Autodesk Inventor part; units mm, degrees
(part 3 of 8)
sketch "20" plane through (0, 0, 0) normal (0, 0, 1) x (1, 0, 0)
  line L0 (110.47, 0) -> (110.47, 86.411)
  line L1 (110.47, 86.411) -> (0, 86.411)
  line L2 (0, 86.411) -> (0, 0)
  line L3 (-2.54, 0) -> (-10.84, 0)
  arc A0 (-10.84, 0.0325) -> (-10.84, -0.0325) centre (-10.84, 0) ccw
  arc A1 (-2.54, -0.0325) -> (-2.54, 0.0325) centre (-2.54, 0) ccw
  line L4 (-2.54, 85.09) -> (-10.84, 85.09)
  arc A2 (-10.84, 85.1225) -> (-10.84, 85.0575) centre (-10.84, 85.09) ccw
  arc A3 (-2.54, 85.0575) -> (-2.54, 85.1225) centre (-2.54, 85.09) ccw
  line L5 (-8.89, 0.065) -> (-8.89, 85.025)
  arc A4 (-8.8575, 85.025) -> (-8.9225, 85.025) centre (-8.89, 85.025) ccw
  arc A5 (-8.9225, 0.065) -> (-8.8575, 0.065) centre (-8.89, 0.065) ccw
  line L6 (-8.89, 0.065) -> (-9.2092, 2.6)
  arc A6 (-9.177, 2.6041) -> (-9.2415, 2.5959) centre (-9.2093, 2.6) ccw
  arc A7 (-8.9222, 0.0609) -> (-8.8578, 0.0691) centre (-8.89, 0.065) ccw
  line L7 (-9.2092, 2.6) -> (-8.5708, 2.6)
  arc A8 (-8.5708, 2.5675) -> (-8.5708, 2.6325) centre (-8.5708, 2.6) ccw
  arc A9 (-9.2092, 2.6325) -> (-9.2092, 2.5675) centre (-9.2092, 2.6) ccw
  line L8 (-8.5708, 2.6) -> (-8.89, 0.065)
  arc A10 (-8.9222, 0.0691) -> (-8.8578, 0.0609) centre (-8.89, 0.065) ccw
  arc A11 (-8.5385, 2.5959) -> (-8.603, 2.6041) centre (-8.5707, 2.6) ccw
  line L9 (-8.89, 0.065) -> (-9.02, 2.6)
  arc A12 (-8.9875, 2.6017) -> (-9.0525, 2.5983) centre (-9.02, 2.6) ccw
  arc A13 (-8.9225, 0.0633) -> (-8.8575, 0.0667) centre (-8.89, 0.065) ccw
  line L10 (-8.76, 2.6) -> (-8.89, 0.065)
  arc A14 (-8.9225, 0.0667) -> (-8.8575, 0.0633) centre (-8.89, 0.065) ccw
  arc A15 (-8.7275, 2.5983) -> (-8.7925, 2.6017) centre (-8.76, 2.6) ccw
  line L11 (-8.89, 0.065) -> (-9.15, 2.6)
  arc A16 (-9.1177, 2.6033) -> (-9.1823, 2.5967) centre (-9.15, 2.6) ccw
  arc A17 (-8.9223, 0.0617) -> (-8.8577, 0.0683) centre (-8.89, 0.065) ccw
  line L12 (-8.63, 2.6) -> (-8.89, 0.065)
  arc A18 (-8.9223, 0.0683) -> (-8.8577, 0.0617) centre (-8.89, 0.065) ccw
  arc A19 (-8.5977, 2.5967) -> (-8.6623, 2.6033) centre (-8.63, 2.6) ccw
  line L13 (-8.89, 85.025) -> (-9.2092, 82.49)
  arc A20 (-9.2415, 82.4941) -> (-9.177, 82.4859) centre (-9.2093, 82.49) ccw
  arc A21 (-8.8578, 85.0209) -> (-8.9222, 85.0291) centre (-8.89, 85.025) ccw
  line L14 (-9.2092, 82.49) -> (-8.5708, 82.49)
  arc A22 (-8.5708, 82.4575) -> (-8.5708, 82.5225) centre (-8.5708, 82.49) ccw
  arc A23 (-9.2092, 82.5225) -> (-9.2092, 82.4575) centre (-9.2092, 82.49) ccw
  line L15 (-8.5708, 82.49) -> (-8.89, 85.025)
  arc A24 (-8.8578, 85.0291) -> (-8.9222, 85.0209) centre (-8.89, 85.025) ccw
  arc A25 (-8.603, 82.4859) -> (-8.5385, 82.4941) centre (-8.5707, 82.49) ccw
  line L16 (-8.89, 85.025) -> (-9.02, 82.49)
  arc A26 (-9.0525, 82.4917) -> (-8.9875, 82.4883) centre (-9.02, 82.49) ccw
  arc A27 (-8.8575, 85.0233) -> (-8.9225, 85.0267) centre (-8.89, 85.025) ccw
  line L17 (-8.76, 82.49) -> (-8.89, 85.025)
  arc A28 (-8.8575, 85.0267) -> (-8.9225, 85.0233) centre (-8.89, 85.025) ccw
  arc A29 (-8.7925, 82.4883) -> (-8.7275, 82.4917) centre (-8.76, 82.49) ccw
  line L18 (-8.89, 85.025) -> (-9.15, 82.49)
  arc A30 (-9.1823, 82.4933) -> (-9.1177, 82.4867) centre (-9.15, 82.49) ccw
  arc A31 (-8.8577, 85.0217) -> (-8.9223, 85.0283) centre (-8.89, 85.025) ccw
  line L19 (-8.63, 82.49) -> (-8.89, 85.025)
  arc A32 (-8.8577, 85.0283) -> (-8.9223, 85.0217) centre (-8.89, 85.025) ccw
  arc A33 (-8.6623, 82.4867) -> (-8.5977, 82.4933) centre (-8.63, 82.49) ccw
  arc A34 (-9.9923, 40.3333) -> (-9.9923, 39.4302) centre (-9.9923, 39.8817) ccw
  arc A35 (-9.9923, 40.2952) -> (-9.9923, 40.3714) centre (-9.9923, 40.3333) ccw
  arc A36 (-9.9923, 39.3921) -> (-9.9923, 39.4683) centre (-9.9923, 39.4302) ccw
  arc A37 (-9.9923, 39.4302) -> (-9.9923, 40.3333) centre (-9.9923, 39.8817) ccw
  arc A38 (-9.9923, 39.4683) -> (-9.9923, 39.3921) centre (-9.9923, 39.4302) ccw
  arc A39 (-9.9923, 40.3714) -> (-9.9923, 40.2952) centre (-9.9923, 40.3333) ccw
  arc A40 (-10.8051, 40.243) -> (-10.8051, 39.5205) centre (-10.8051, 39.8817) ccw
  arc A41 (-10.8051, 40.2049) -> (-10.8051, 40.2811) centre (-10.8051, 40.243) ccw
  arc A42 (-10.8051, 39.4824) -> (-10.8051, 39.5586) centre (-10.8051, 39.5205) ccw
  arc A43 (-10.8051, 39.5205) -> (-10.8051, 40.243) centre (-10.8051, 39.8817) ccw
  arc A44 (-10.8051, 39.5586) -> (-10.8051, 39.4824) centre (-10.8051, 39.5205) ccw
  arc A45 (-10.8051, 40.2811) -> (-10.8051, 40.2049) centre (-10.8051, 40.243) ccw
  line L20 (-9.5407, 40.9933) -> (-9.5407, 41.5352)
  arc A46 (-9.5026, 41.5352) -> (-9.5788, 41.5352) centre (-9.5407, 41.5352) ccw
  arc A47 (-9.5788, 40.9933) -> (-9.5026, 40.9933) centre (-9.5407, 40.9933) ccw
  arc A48 (-9.5407, 41.5352) -> (-9.9019, 41.8964) centre (-9.9019, 41.5352) ccw
  arc A49 (-9.5788, 41.5352) -> (-9.5026, 41.5352) centre (-9.5407, 41.5352) ccw
  arc A50 (-9.9019, 41.9345) -> (-9.9019, 41.8583) centre (-9.9019, 41.8964) ccw
  line L21 (-9.9019, 41.8964) -> (-10.0826, 41.8964)
  arc A51 (-10.0826, 41.9345) -> (-10.0826, 41.8583) centre (-10.0826, 41.8964) ccw
  arc A52 (-9.9019, 41.8583) -> (-9.9019, 41.9345) centre (-9.9019, 41.8964) ccw
  arc A53 (-10.0826, 41.8964) -> (-10.4438, 41.5352) centre (-10.0826, 41.5352) ccw
  arc A54 (-10.0826, 41.8583) -> (-10.0826, 41.9345) centre (-10.0826, 41.8964) ccw
  line L22 (110.425, 90.17) -> (107.89, 90.43)
  arc A55 (107.8883, 90.0725) -> (107.8917, 90.0075) centre (107.89, 90.04) ccw
  arc A56 (110.4267, 90.1375) -> (110.4233, 90.2025) centre (110.425, 90.17) ccw
  line L23 (107.89, 90.04) -> (110.425, 90.17)
  arc A57 (110.4233, 90.1375) -> (110.4267, 90.2025) centre (110.425, 90.17) ccw
  arc A58 (107.8917, 90.3325) -> (107.8883, 90.2675) centre (107.89, 90.3) ccw
  line L24 (110.425, 90.17) -> (107.89, 90.3)
  arc A59 (107.8859, 89.883) -> (107.8941, 89.8185) centre (107.89, 89.8507) ccw
  arc A60 (110.4291, 90.1378) -> (110.4209, 90.2022) centre (110.425, 90.17) ccw
  line L25 (107.89, 89.8508) -> (110.425, 90.17)
  arc A61 (58.3921, 91.9044) -> (58.7533, 91.5432) centre (58.7533, 91.9044) ccw
  arc A62 (59.2952, 91.5051) -> (59.2952, 91.5813) centre (59.2952, 91.5432) ccw
  arc A63 (58.7533, 91.5813) -> (58.7533, 91.5051) centre (58.7533, 91.5432) ccw
  line L26 (59.2952, 91.5432) -> (58.7533, 91.5432)
  arc A64 (2.6325, 90.4892) -> (2.5675, 90.4892) centre (2.6, 90.4892) ccw
  arc A65 (2.5675, 89.8508) -> (2.6325, 89.8508) centre (2.6, 89.8508) ccw
  line L27 (2.6, 90.4892) -> (2.6, 89.8508)
  arc A66 (0.0609, 90.2022) -> (0.0691, 90.1378) centre (0.065, 90.17) ccw
  arc A67 (2.6041, 90.457) -> (2.5959, 90.5215) centre (2.6, 90.4893) ccw
  line L28 (0.065, 90.17) -> (2.6, 90.4892)
  arc A68 (0.065, 90.2025) -> (0.065, 90.1375) centre (0.065, 90.17) ccw
  arc A69 (110.425, 90.1375) -> (110.425, 90.2025) centre (110.425, 90.17) ccw
  line L29 (0.065, 90.17) -> (110.425, 90.17)
  arc A70 (110.4575, 87.63) -> (110.5225, 87.63) centre (110.49, 87.63) ccw
  arc A71 (110.5225, 92.12) -> (110.4575, 92.12) centre (110.49, 92.12) ccw
  line L30 (110.49, 87.63) -> (110.49, 92.12)
  arc A72 (57.4992, 91.5432) -> (57.423, 91.5432) centre (57.4611, 91.5432) ccw
  arc A73 (57.423, 90.8207) -> (57.4992, 90.8207) centre (57.4611, 90.8207) ccw
  line L31 (57.4611, 91.5432) -> (57.4611, 90.8207)
  arc A74 (56.8289, 91.22) -> (56.8289, 91.1438) centre (56.8289, 91.1819) ccw
  arc A75 (57.732, 91.1438) -> (57.732, 91.22) centre (57.732, 91.1819) ccw
  line L32 (56.8289, 91.1819) -> (57.732, 91.1819)
  arc A76 (57.2268, 92.4358) -> (57.1535, 92.4568) centre (57.1902, 92.4463) ccw
  arc A77 (56.7923, 91.1924) -> (56.8656, 91.1715) centre (56.829, 91.182) ccw
  line L33 (59.2952, 91.9947) -> (59.2952, 91.5432)
  arc A78 (58.354, 91.9947) -> (58.4302, 91.9947) centre (58.3921, 91.9947) ccw
  arc A79 (59.2571, 91.9947) -> (59.3333, 91.9947) centre (59.2952, 91.9947) ccw
  arc A80 (107.8575, 89.8508) -> (107.9225, 89.8508) centre (107.89, 89.8508) ccw
  arc A81 (59.2952, 91.9947) -> (58.3921, 91.9947) centre (58.8436, 91.9947) ccw
  arc A82 (58.354, 91.9044) -> (58.4302, 91.9044) centre (58.3921, 91.9044) ccw
  arc A83 (58.4302, 91.9947) -> (58.354, 91.9947) centre (58.3921, 91.9947) ccw
  circle A84 centre (87.376, 65.7225) radius 1.524
  circle A85 centre (87.376, 19.431) radius 1.524
  circle A86 centre (22.225, 19.431) radius 1.524
  line L34 (57.1902, 92.4463) -> (56.8289, 91.1819)
  arc A87 (56.2315, 90.7826) -> (56.2315, 90.8588) centre (56.2315, 90.8207) ccw
  arc A88 (56.1411, 90.8588) -> (56.1411, 90.7826) centre (56.1411, 90.8207) ccw
  arc A89 (-0.0325, 87.63) -> (0.0325, 87.63) centre (0, 87.63) ccw
  arc A90 (0.0325, 92.12) -> (-0.0325, 92.12) centre (0, 92.12) ccw
  line L35 (0, 87.63) -> (0, 92.12)
  arc A91 (-10.2632, 45.686) -> (-10.2632, 45.6098) centre (-10.2632, 45.6479) ccw
  arc A92 (-9.5788, 44.9254) -> (-9.5026, 44.9254) centre (-9.5407, 44.9254) ccw
  arc A93 (-9.5407, 44.9254) -> (-10.2632, 45.6479) centre (-10.2632, 44.9254) ccw
  arc A94 (-10.7147, 45.686) -> (-10.7147, 45.6098) centre (-10.7147, 45.6479) ccw
  arc A95 (-10.2632, 45.6098) -> (-10.2632, 45.686) centre (-10.2632, 45.6479) ccw
  line L36 (-10.7147, 45.6479) -> (-10.2632, 45.6479)
  line L37 (56.2315, 90.8207) -> (56.1411, 90.8207)
  arc A96 (56.2696, 90.911) -> (56.1934, 90.911) centre (56.2315, 90.911) ccw
  arc A97 (56.1934, 90.8207) -> (56.2696, 90.8207) centre (56.2315, 90.8207) ccw
  line L38 (56.2315, 90.911) -> (56.2315, 90.8207)
  arc A98 (56.1411, 90.9491) -> (56.1411, 90.8729) centre (56.1411, 90.911) ccw
  arc A99 (56.2315, 90.8729) -> (56.2315, 90.9491) centre (56.2315, 90.911) ccw
  line L39 (56.1411, 90.911) -> (56.2315, 90.911)
  arc A100 (56.103, 90.8207) -> (56.1792, 90.8207) centre (56.1411, 90.8207) ccw
  arc A101 (56.1792, 90.911) -> (56.103, 90.911) centre (56.1411, 90.911) ccw
  line L40 (56.1411, 90.8207) -> (56.1411, 90.911)
  circle A102 centre (22.225, 65.7225) radius 1.524
  arc A103 (59.3333, 91.5432) -> (59.2571, 91.5432) centre (59.2952, 91.5432) ccw
  arc A104 (58.5727, 90.8588) -> (58.5727, 90.7826) centre (58.5727, 90.8207) ccw
  arc A105 (58.5727, 90.8207) -> (59.2952, 91.5432) centre (58.5727, 91.5432) ccw
  arc A106 (59.3333, 91.9947) -> (59.2571, 91.9947) centre (59.2952, 91.9947) ccw
  arc A107 (59.2571, 91.5432) -> (59.3333, 91.5432) centre (59.2952, 91.5432) ccw
  arc A108 (54.7011, 91.2057) -> (54.7606, 91.1581) centre (54.7309, 91.1819) ccw
  arc A109 (55.4831, 92.0613) -> (55.4236, 92.1089) centre (55.4534, 92.0851) ccw
  line L41 (54.7309, 91.1819) -> (55.4534, 92.0851)
  arc A110 (55.4442, 91.0341) -> (55.3722, 91.0588) centre (55.4082, 91.0464) ccw
  arc A111 (55.0921, 90.8588) -> (55.0921, 90.7826) centre (55.0921, 90.8207) ccw
  arc A112 (55.0921, 90.8207) -> (55.4082, 91.0465) centre (55.0921, 91.1548) ccw
  arc A113 (55.5818, 91.6335) -> (55.5056, 91.6335) centre (55.5437, 91.6335) ccw
  arc A114 (55.374, 91.0632) -> (55.4425, 91.0298) centre (55.4083, 91.0465) ccw
  arc A115 (55.4082, 91.0465) -> (55.5437, 91.6335) centre (54.2043, 91.6336) ccw
  arc A116 (55.0921, 90.7826) -> (55.0921, 90.8588) centre (55.0921, 90.8207) ccw
  arc A117 (54.8121, 91.0588) -> (54.74, 91.0341) centre (54.7761, 91.0464) ccw
  arc A118 (54.776, 91.0465) -> (55.0921, 90.8207) centre (55.0921, 91.1548) ccw
  arc A119 (54.7418, 91.0298) -> (54.8103, 91.0632) centre (54.7761, 91.0465) ccw
  arc A120 (54.6787, 91.6335) -> (54.6025, 91.6335) centre (54.6406, 91.6335) ccw
  arc A121 (54.6406, 91.6335) -> (54.776, 91.0465) centre (55.98, 91.6333) ccw
  arc A122 (55.4425, 92.2372) -> (55.374, 92.2038) centre (55.4083, 92.2205) ccw
  arc A123 (55.5056, 91.6335) -> (55.5818, 91.6335) centre (55.5437, 91.6335) ccw
  arc A124 (55.5437, 91.6335) -> (55.4082, 92.2205) centre (54.2043, 91.6334) ccw
  arc A125 (55.0921, 92.4844) -> (55.0921, 92.4082) centre (55.0921, 92.4463) ccw
  arc A126 (55.3722, 92.2082) -> (55.4442, 92.2329) centre (55.4082, 92.2206) ccw
  line L42 (0, 0) -> (110.47, 0)
  arc A127 (55.4082, 92.2205) -> (55.0921, 92.4463) centre (55.0921, 92.1122) ccw
  arc A128 (54.74, 92.2329) -> (54.8121, 92.2082) centre (54.7761, 92.2206) ccw
  arc A129 (55.0921, 92.4082) -> (55.0921, 92.4844) centre (55.0921, 92.4463) ccw
  arc A130 (55.0921, 92.4463) -> (54.776, 92.2205) centre (55.0921, 92.1122) ccw
  arc A131 (54.6025, 91.6335) -> (54.6787, 91.6335) centre (54.6406, 91.6335) ccw
  arc A132 (54.8103, 92.2038) -> (54.7418, 92.2372) centre (54.7761, 92.2205) ccw
  arc A133 (54.776, 92.2205) -> (54.6406, 91.6335) centre (55.98, 91.6337) ccw
  arc A134 (53.0774, 90.8588) -> (53.0774, 90.7826) centre (53.0774, 90.8207) ccw
  arc A135 (53.9805, 90.7826) -> (53.9805, 90.8588) centre (53.9805, 90.8207) ccw
  line L43 (53.0774, 90.8207) -> (53.9805, 90.8207)
  line L44 (107.89, 90.4892) -> (107.89, 89.8508)
  arc A136 (110.4209, 90.1378) -> (110.4291, 90.2022) centre (110.425, 90.17) ccw
  arc A137 (107.8941, 90.5215) -> (107.8859, 90.457) centre (107.89, 90.4893) ccw
  line L45 (110.425, 90.17) -> (107.89, 90.4892)
  arc A138 (2.5967, 89.8777) -> (2.6033, 89.9423) centre (2.6, 89.91) ccw
  arc A139 (0.0683, 90.2023) -> (0.0617, 90.1377) centre (0.065, 90.17) ccw
  line L46 (2.6, 89.91) -> (0.065, 90.17)
  arc A140 (0.0617, 90.2023) -> (0.0683, 90.1377) centre (0.065, 90.17) ccw
  arc A141 (2.6033, 90.3977) -> (2.5967, 90.4623) centre (2.6, 90.43) ccw
  line L47 (0.065, 90.17) -> (2.6, 90.43)
  arc A142 (2.5983, 90.0075) -> (2.6017, 90.0725) centre (2.6, 90.04) ccw
  arc A143 (0.0667, 90.2025) -> (0.0633, 90.1375) centre (0.065, 90.17) ccw
  line L48 (2.6, 90.04) -> (0.065, 90.17)
  arc A144 (0.0633, 90.2025) -> (0.0667, 90.1375) centre (0.065, 90.17) ccw
  arc A145 (2.6017, 90.2675) -> (2.5983, 90.3325) centre (2.6, 90.3) ccw
  line L49 (0.065, 90.17) -> (2.6, 90.3)
  arc A146 (2.5959, 89.8185) -> (2.6041, 89.883) centre (2.6, 89.8507) ccw
  arc A147 (0.0691, 90.2022) -> (0.0609, 90.1378) centre (0.065, 90.17) ccw
  arc A148 (53.5671, 92.4463) -> (53.4909, 92.4463) centre (53.529, 92.4463) ccw
  arc A149 (53.4909, 90.8207) -> (53.5671, 90.8207) centre (53.529, 90.8207) ccw
  line L50 (53.529, 92.4463) -> (53.529, 90.8207)
  line L51 (2.6, 89.8508) -> (0.065, 90.17)
  arc A150 (53.0536, 92.1148) -> (53.1012, 92.0553) centre (53.0774, 92.0851) ccw
  arc A151 (53.5528, 92.4165) -> (53.5052, 92.4761) centre (53.529, 92.4463) ccw
  line L52 (53.0774, 92.0851) -> (53.529, 92.4463)
  arc A152 (51.5143, 90.8588) -> (51.5143, 90.7826) centre (51.5143, 90.8207) ccw
  arc A153 (52.4174, 90.7826) -> (52.4174, 90.8588) centre (52.4174, 90.8207) ccw
  line L53 (51.5143, 90.8207) -> (52.4174, 90.8207)
  arc A154 (52.004, 92.4463) -> (51.9278, 92.4463) centre (51.9659, 92.4463) ccw
  arc A155 (107.9225, 90.4892) -> (107.8575, 90.4892) centre (107.89, 90.4892) ccw
  arc A156 (51.9278, 90.8207) -> (52.004, 90.8207) centre (51.9659, 90.8207) ccw
  line L54 (51.9659, 92.4463) -> (51.9659, 90.8207)
  arc A157 (51.4905, 92.1148) -> (51.5381, 92.0553) centre (51.5143, 92.0851) ccw
  arc A158 (51.9897, 92.4165) -> (51.9421, 92.4761) centre (51.9659, 92.4463) ccw
  line L55 (51.5143, 92.0851) -> (51.9659, 92.4463)
  arc A159 (107.8867, 89.9423) -> (107.8933, 89.8777) centre (107.89, 89.91) ccw
  arc A160 (110.4283, 90.1377) -> (110.4217, 90.2023) centre (110.425, 90.17) ccw
  line L56 (58.3921, 91.9044) -> (58.3921, 91.9947)
  arc A161 (58.7533, 91.5051) -> (58.7533, 91.5813) centre (58.7533, 91.5432) ccw
  arc A162 (58.4302, 91.9044) -> (58.354, 91.9044) centre (58.3921, 91.9044) ccw
  line L57 (107.89, 89.91) -> (110.425, 90.17)
  arc A163 (110.4217, 90.1377) -> (110.4283, 90.2023) centre (110.425, 90.17) ccw
  arc A164 (-10.7147, 44.7067) -> (-10.7147, 44.7829) centre (-10.7147, 44.7448) ccw
  arc A165 (-10.7147, 45.6098) -> (-10.7147, 45.686) centre (-10.7147, 45.6479) ccw
  arc A166 (-10.7147, 45.6479) -> (-10.7147, 44.7448) centre (-10.7147, 45.1964) ccw
  arc A167 (-10.6244, 44.7067) -> (-10.6244, 44.7829) centre (-10.6244, 44.7448) ccw
  arc A168 (-10.7147, 44.7829) -> (-10.7147, 44.7067) centre (-10.7147, 44.7448) ccw
  line L58 (-10.6244, 44.7448) -> (-10.7147, 44.7448)
  arc A169 (-10.2251, 45.1061) -> (-10.3013, 45.1061) centre (-10.2632, 45.1061) ccw
  arc A170 (-10.6244, 44.7829) -> (-10.6244, 44.7067) centre (-10.6244, 44.7448) ccw
  arc A171 (-10.6244, 44.7448) -> (-10.2632, 45.1061) centre (-10.6245, 45.1061) ccw
  arc A172 (-10.2251, 45.6479) -> (-10.3013, 45.6479) centre (-10.2632, 45.6479) ccw
  arc A173 (-10.3013, 45.1061) -> (-10.2251, 45.1061) centre (-10.2632, 45.1061) ccw
  line L59 (-10.2632, 45.6479) -> (-10.2632, 45.1061)
  arc A174 (-9.9257, 43.2422) -> (-9.8781, 43.3018) centre (-9.9019, 43.272) ccw
  arc A175 (-10.7813, 44.0242) -> (-10.8289, 43.9647) centre (-10.8051, 43.9945) ccw
  line L60 (-9.9019, 43.272) -> (-10.8051, 43.9945)
  arc A176 (-9.7541, 43.9854) -> (-9.7788, 43.9133) centre (-9.7664, 43.9493) ccw
  arc A177 (-9.5788, 43.6332) -> (-9.5026, 43.6332) centre (-9.5407, 43.6332) ccw
  arc A178 (-9.5407, 43.6332) -> (-9.7665, 43.9493) centre (-9.8748, 43.6332) ccw
  arc A179 (-10.3535, 44.1229) -> (-10.3535, 44.0467) centre (-10.3535, 44.0848) ccw
  arc A180 (-9.7832, 43.9151) -> (-9.7498, 43.9836) centre (-9.7665, 43.9494) ccw
  arc A181 (-9.7665, 43.9493) -> (-10.3535, 44.0848) centre (-10.3536, 42.7454) ccw
  arc A182 (-9.5026, 43.6332) -> (-9.5788, 43.6332) centre (-9.5407, 43.6332) ccw
  arc A183 (-9.7788, 43.3532) -> (-9.7541, 43.2811) centre (-9.7664, 43.3171) ccw
  arc A184 (-9.7665, 43.3172) -> (-9.5407, 43.6332) centre (-9.8748, 43.6332) ccw
  arc A185 (-9.7498, 43.2829) -> (-9.7832, 43.3514) centre (-9.7665, 43.3171) ccw
  arc A186 (-10.3535, 43.2198) -> (-10.3535, 43.1436) centre (-10.3535, 43.1817) ccw
  arc A187 (-10.3535, 43.1817) -> (-9.7665, 43.3172) centre (-10.3536, 44.5211) ccw
  arc A188 (-10.9572, 43.9836) -> (-10.9238, 43.9151) centre (-10.9405, 43.9494) ccw
  arc A189 (-10.3535, 44.0467) -> (-10.3535, 44.1229) centre (-10.3535, 44.0848) ccw
  arc A190 (-10.3535, 44.0848) -> (-10.9405, 43.9493) centre (-10.3534, 42.7454) ccw
  arc A191 (-11.2044, 43.6332) -> (-11.1282, 43.6332) centre (-11.1663, 43.6332) ccw
  arc A192 (-10.9282, 43.9133) -> (-10.9529, 43.9854) centre (-10.9405, 43.9493) ccw
  arc A193 (-10.9405, 43.9493) -> (-11.1663, 43.6332) centre (-10.8322, 43.6332) ccw
  arc A194 (-10.9529, 43.2811) -> (-10.9282, 43.3532) centre (-10.9405, 43.3171) ccw
  arc A195 (-11.1282, 43.6332) -> (-11.2044, 43.6332) centre (-11.1663, 43.6332) ccw
  arc A196 (-11.1663, 43.6332) -> (-10.9405, 43.3172) centre (-10.8322, 43.6332) ccw
  arc A197 (-10.3535, 43.1436) -> (-10.3535, 43.2198) centre (-10.3535, 43.1817) ccw
  arc A198 (-10.9238, 43.3514) -> (-10.9572, 43.2829) centre (-10.9405, 43.3171) ccw
  arc A199 (-10.9405, 43.3172) -> (-10.3535, 43.1817) centre (-10.3534, 44.5211) ccw
  arc A200 (-9.5026, 42.5842) -> (-9.5788, 42.5842) centre (-9.5407, 42.5842) ccw
  arc A201 (-9.5788, 42.4939) -> (-9.5026, 42.4939) centre (-9.5407, 42.4939) ccw
  line L61 (-9.5407, 42.5842) -> (-9.5407, 42.4939)
  arc A202 (-9.631, 42.6223) -> (-9.631, 42.5461) centre (-9.631, 42.5842) ccw
  arc A203 (-9.5407, 42.5461) -> (-9.5407, 42.6223) centre (-9.5407, 42.5842) ccw
  line L62 (-9.631, 42.5842) -> (-9.5407, 42.5842)
  arc A204 (-9.6691, 42.4939) -> (-9.5929, 42.4939) centre (-9.631, 42.4939) ccw
  arc A205 (-9.5929, 42.5842) -> (-9.6691, 42.5842) centre (-9.631, 42.5842) ccw
  line L63 (-9.631, 42.4939) -> (-9.631, 42.5842)
  arc A206 (-9.5407, 42.4558) -> (-9.5407, 42.532) centre (-9.5407, 42.4939) ccw
  arc A207 (-9.631, 42.532) -> (-9.631, 42.4558) centre (-9.631, 42.4939) ccw
  line L64 (-9.5407, 42.4939) -> (-9.631, 42.4939)
  arc A208 (-11.2044, 40.9933) -> (-11.1282, 40.9933) centre (-11.1663, 40.9933) ccw
  arc A209 (-11.1282, 41.8964) -> (-11.2044, 41.8964) centre (-11.1663, 41.8964) ccw
  line L65 (-11.1663, 40.9933) -> (-11.1663, 41.8964)
  arc A210 (-10.4438, 40.9552) -> (-10.4438, 41.0314) centre (-10.4438, 40.9933) ccw
  arc A211 (-11.1663, 41.0314) -> (-11.1663, 40.9552) centre (-11.1663, 40.9933) ccw
  line L66 (-10.4438, 40.9933) -> (-11.1663, 40.9933)
  arc A212 (-10.4057, 41.5352) -> (-10.4819, 41.5352) centre (-10.4438, 41.5352) ccw
  arc A213 (-10.4819, 40.9933) -> (-10.4057, 40.9933) centre (-10.4438, 40.9933) ccw
  line L67 (-10.4438, 41.5352) -> (-10.4438, 40.9933)
  arc A214 (-10.4819, 41.5352) -> (-10.4057, 41.5352) centre (-10.4438, 41.5352) ccw
  arc A215 (107.8933, 90.4623) -> (107.8867, 90.3977) centre (107.89, 90.43) ccw
  constraints: 514 point on circle, 216 centre point, 136 end point, 44 point on line, 2 midpoint
sketch "21" plane through (0, 0, 0) normal (0, 0, 1) x (1, 0, 0)
  line L0 (81.6034, 53.0011) -> (81.3946, 53.0011)
  arc A0 (81.3946, 53.0202) -> (81.3946, 52.9821) centre (81.3946, 53.0012) ccw
  arc A1 (81.6034, 52.9821) -> (81.6034, 53.0202) centre (81.6034, 53.0012) ccw
  line L1 (81.499, 55.4188) -> (81.2902, 54.6879)
  arc A2 (81.2719, 54.6931) -> (81.3085, 54.6826) centre (81.2902, 54.6879) ccw
  arc A3 (81.5173, 55.4136) -> (81.4807, 55.424) centre (81.499, 55.4188) ccw
  line L2 (81.2902, 54.6879) -> (81.8123, 54.6879)
  arc A4 (81.8123, 54.6688) -> (81.8123, 54.7069) centre (81.8123, 54.6879) ccw
  arc A5 (81.2902, 54.7069) -> (81.2902, 54.6688) centre (81.2902, 54.6879) ccw
  line L3 (81.6557, 54.8967) -> (81.6557, 54.479)
  arc A6 (81.6366, 54.479) -> (81.6747, 54.479) centre (81.6557, 54.479) ccw
  arc A7 (81.6747, 54.8967) -> (81.6366, 54.8967) centre (81.6557, 54.8967) ccw
  arc A8 (76.8504, 45.9569) -> (76.8504, 61.9569) centre (76.8504, 53.9569) ccw
  arc A9 (76.8504, 61.9569) -> (76.8504, 45.9569) centre (76.8504, 53.9569) ccw
  arc A10 (76.8504, 47.4377) -> (76.8504, 60.4761) centre (76.8504, 53.9569) ccw
  arc A11 (76.8504, 60.4761) -> (76.8504, 47.4377) centre (76.8504, 53.9569) ccw
  arc A12 (76.8504, 44.4569) -> (76.8504, 63.4569) centre (76.8504, 53.9569) ccw
  arc A13 (76.8504, 63.4569) -> (76.8504, 44.4569) centre (76.8504, 53.9569) ccw
  line L4 (24.13, 24.13) -> (24.13, 26.67)
  arc A14 (24.1681, 26.67) -> (24.0919, 26.67) centre (24.13, 26.67) ccw
  arc A15 (24.0919, 24.13) -> (24.1681, 24.13) centre (24.13, 24.13) ccw
  line L5 (24.13, 26.67) -> (21.844, 26.67)
  arc A16 (21.844, 26.7081) -> (21.844, 26.6319) centre (21.844, 26.67) ccw
  arc A17 (24.13, 26.6319) -> (24.13, 26.7081) centre (24.13, 26.67) ccw
  line L6 (21.844, 26.67) -> (21.59, 26.416)
  arc A18 (21.5631, 26.4429) -> (21.6169, 26.3891) centre (21.59, 26.416) ccw
  arc A19 (21.8709, 26.6431) -> (21.8171, 26.6969) centre (21.844, 26.67) ccw
  line L7 (21.59, 26.416) -> (21.336, 26.67)
  arc A20 (21.3629, 26.6969) -> (21.3091, 26.6431) centre (21.336, 26.67) ccw
  arc A21 (21.5631, 26.3891) -> (21.6169, 26.4429) centre (21.59, 26.416) ccw
  line L8 (21.336, 26.67) -> (19.304, 26.67)
  arc A22 (19.304, 26.7081) -> (19.304, 26.6319) centre (19.304, 26.67) ccw
  arc A23 (21.336, 26.6319) -> (21.336, 26.7081) centre (21.336, 26.67) ccw
  line L9 (19.304, 26.67) -> (19.05, 26.416)
  arc A24 (19.0231, 26.4429) -> (19.0769, 26.3891) centre (19.05, 26.416) ccw
  arc A25 (19.3309, 26.6431) -> (19.2771, 26.6969) centre (19.304, 26.67) ccw
  line L10 (19.05, 26.416) -> (18.796, 26.67)
  arc A26 (18.8229, 26.6969) -> (18.7691, 26.6431) centre (18.796, 26.67) ccw
  arc A27 (19.0231, 26.3891) -> (19.0769, 26.4429) centre (19.05, 26.416) ccw
  line L11 (18.796, 26.67) -> (16.764, 26.67)
  arc A28 (16.764, 26.7081) -> (16.764, 26.6319) centre (16.764, 26.67) ccw
  arc A29 (18.796, 26.6319) -> (18.796, 26.7081) centre (18.796, 26.67) ccw
  line L12 (16.764, 26.67) -> (16.51, 26.416)
  arc A30 (16.4831, 26.4429) -> (16.5369, 26.3891) centre (16.51, 26.416) ccw
  arc A31 (16.7909, 26.6431) -> (16.7371, 26.6969) centre (16.764, 26.67) ccw
  line L13 (16.51, 26.416) -> (16.256, 26.67)
  arc A32 (16.2829, 26.6969) -> (16.2291, 26.6431) centre (16.256, 26.67) ccw
  arc A33 (16.4831, 26.3891) -> (16.5369, 26.4429) centre (16.51, 26.416) ccw
  line L14 (16.256, 26.67) -> (14.224, 26.67)
  arc A34 (14.224, 26.7081) -> (14.224, 26.6319) centre (14.224, 26.67) ccw
  arc A35 (16.256, 26.6319) -> (16.256, 26.7081) centre (16.256, 26.67) ccw
  line L15 (14.224, 26.67) -> (13.97, 26.416)
  arc A36 (13.9431, 26.4429) -> (13.9969, 26.3891) centre (13.97, 26.416) ccw
  arc A37 (14.2509, 26.6431) -> (14.1971, 26.6969) centre (14.224, 26.67) ccw
  line L16 (13.97, 26.416) -> (13.716, 26.67)
  arc A38 (13.7429, 26.6969) -> (13.6891, 26.6431) centre (13.716, 26.67) ccw
  arc A39 (13.9431, 26.3891) -> (13.9969, 26.4429) centre (13.97, 26.416) ccw
  line L17 (6.35, 26.67) -> (6.35, 24.13)
  arc A40 (6.3119, 24.13) -> (6.3881, 24.13) centre (6.35, 24.13) ccw
  arc A41 (6.3881, 26.67) -> (6.3119, 26.67) centre (6.35, 26.67) ccw
  line L18 (13.716, 24.13) -> (13.97, 24.384)
  arc A42 (13.9969, 24.3571) -> (13.9431, 24.4109) centre (13.97, 24.384) ccw
  arc A43 (13.6891, 24.1569) -> (13.7429, 24.1031) centre (13.716, 24.13) ccw
  line L19 (13.97, 24.384) -> (14.224, 24.13)
  arc A44 (14.1971, 24.1031) -> (14.2509, 24.1569) centre (14.224, 24.13) ccw
  arc A45 (13.9969, 24.4109) -> (13.9431, 24.3571) centre (13.97, 24.384) ccw
  line L20 (14.224, 24.13) -> (16.256, 24.13)
  arc A46 (16.256, 24.0919) -> (16.256, 24.1681) centre (16.256, 24.13) ccw
  arc A47 (14.224, 24.1681) -> (14.224, 24.0919) centre (14.224, 24.13) ccw
  line L21 (16.256, 24.13) -> (16.51, 24.384)
  arc A48 (16.5369, 24.3571) -> (16.4831, 24.4109) centre (16.51, 24.384) ccw
  arc A49 (16.2291, 24.1569) -> (16.2829, 24.1031) centre (16.256, 24.13) ccw
  line L22 (16.51, 24.384) -> (16.764, 24.13)
  arc A50 (16.7371, 24.1031) -> (16.7909, 24.1569) centre (16.764, 24.13) ccw
  arc A51 (16.5369, 24.4109) -> (16.4831, 24.3571) centre (16.51, 24.384) ccw
  line L23 (16.764, 24.13) -> (18.796, 24.13)
  arc A52 (18.796, 24.0919) -> (18.796, 24.1681) centre (18.796, 24.13) ccw
  arc A53 (16.764, 24.1681) -> (16.764, 24.0919) centre (16.764, 24.13) ccw
  line L24 (18.796, 24.13) -> (19.05, 24.384)
  arc A54 (19.0769, 24.3571) -> (19.0231, 24.4109) centre (19.05, 24.384) ccw
  arc A55 (18.7691, 24.1569) -> (18.8229, 24.1031) centre (18.796, 24.13) ccw
  line L25 (19.05, 24.384) -> (19.304, 24.13)
  arc A56 (19.2771, 24.1031) -> (19.3309, 24.1569) centre (19.304, 24.13) ccw
  arc A57 (19.0769, 24.4109) -> (19.0231, 24.3571) centre (19.05, 24.384) ccw
  line L26 (19.304, 24.13) -> (21.336, 24.13)
  arc A58 (21.336, 24.0919) -> (21.336, 24.1681) centre (21.336, 24.13) ccw
  arc A59 (19.304, 24.1681) -> (19.304, 24.0919) centre (19.304, 24.13) ccw
  line L27 (21.336, 24.13) -> (21.59, 24.384)
  arc A60 (21.6169, 24.3571) -> (21.5631, 24.4109) centre (21.59, 24.384) ccw
  arc A61 (21.3091, 24.1569) -> (21.3629, 24.1031) centre (21.336, 24.13) ccw
  line L28 (21.59, 24.384) -> (21.844, 24.13)
  arc A62 (21.8171, 24.1031) -> (21.8709, 24.1569) centre (21.844, 24.13) ccw
  arc A63 (21.6169, 24.4109) -> (21.5631, 24.3571) centre (21.59, 24.384) ccw
  line L29 (21.844, 24.13) -> (24.13, 24.13)
  arc A64 (24.13, 24.0919) -> (24.13, 24.1681) centre (24.13, 24.13) ccw
  arc A65 (21.844, 24.1681) -> (21.844, 24.0919) centre (21.844, 24.13) ccw
  line L30 (13.716, 26.67) -> (11.684, 26.67)
  arc A66 (11.684, 26.7081) -> (11.684, 26.6319) centre (11.684, 26.67) ccw
  arc A67 (13.716, 26.6319) -> (13.716, 26.7081) centre (13.716, 26.67) ccw
  line L31 (11.684, 26.67) -> (11.43, 26.416)
  arc A68 (11.4031, 26.4429) -> (11.4569, 26.3891) centre (11.43, 26.416) ccw
  arc A69 (11.7109, 26.6431) -> (11.6571, 26.6969) centre (11.684, 26.67) ccw
  line L32 (11.43, 26.416) -> (11.176, 26.67)
  arc A70 (11.2029, 26.6969) -> (11.1491, 26.6431) centre (11.176, 26.67) ccw
  arc A71 (11.4031, 26.3891) -> (11.4569, 26.4429) centre (11.43, 26.416) ccw
  line L33 (11.176, 26.67) -> (9.144, 26.67)
  arc A72 (9.144, 26.7081) -> (9.144, 26.6319) centre (9.144, 26.67) ccw
  arc A73 (11.176, 26.6319) -> (11.176, 26.7081) centre (11.176, 26.67) ccw
  line L34 (9.144, 26.67) -> (8.89, 26.416)
  arc A74 (8.8631, 26.4429) -> (8.9169, 26.3891) centre (8.89, 26.416) ccw
  arc A75 (9.1709, 26.6431) -> (9.1171, 26.6969) centre (9.144, 26.67) ccw
  line L35 (8.89, 26.416) -> (8.636, 26.67)
  arc A76 (8.6629, 26.6969) -> (8.6091, 26.6431) centre (8.636, 26.67) ccw
  arc A77 (8.8631, 26.3891) -> (8.9169, 26.4429) centre (8.89, 26.416) ccw
  line L36 (8.636, 24.13) -> (8.89, 24.384)
  arc A78 (8.9169, 24.3571) -> (8.8631, 24.4109) centre (8.89, 24.384) ccw
  arc A79 (8.6091, 24.1569) -> (8.6629, 24.1031) centre (8.636, 24.13) ccw
  line L37 (8.89, 24.384) -> (9.144, 24.13)
  arc A80 (9.1171, 24.1031) -> (9.1709, 24.1569) centre (9.144, 24.13) ccw
  arc A81 (8.9169, 24.4109) -> (8.8631, 24.3571) centre (8.89, 24.384) ccw
  line L38 (9.144, 24.13) -> (11.176, 24.13)
  arc A82 (11.176, 24.0919) -> (11.176, 24.1681) centre (11.176, 24.13) ccw
  arc A83 (9.144, 24.1681) -> (9.144, 24.0919) centre (9.144, 24.13) ccw
  line L39 (11.176, 24.13) -> (11.43, 24.384)
  arc A84 (11.4569, 24.3571) -> (11.4031, 24.4109) centre (11.43, 24.384) ccw
  arc A85 (11.1491, 24.1569) -> (11.2029, 24.1031) centre (11.176, 24.13) ccw
  line L40 (11.43, 24.384) -> (11.684, 24.13)
  arc A86 (11.6571, 24.1031) -> (11.7109, 24.1569) centre (11.684, 24.13) ccw
  arc A87 (11.4569, 24.4109) -> (11.4031, 24.3571) centre (11.43, 24.384) ccw
  line L41 (11.684, 24.13) -> (13.716, 24.13)
  arc A88 (13.716, 24.0919) -> (13.716, 24.1681) centre (13.716, 24.13) ccw
  arc A89 (11.684, 24.1681) -> (11.684, 24.0919) centre (11.684, 24.13) ccw
  line L42 (6.35, 24.13) -> (8.636, 24.13)
  arc A90 (8.636, 24.0919) -> (8.636, 24.1681) centre (8.636, 24.13) ccw
  arc A91 (6.35, 24.1681) -> (6.35, 24.0919) centre (6.35, 24.13) ccw
  line L43 (8.636, 26.67) -> (6.35, 26.67)
  arc A92 (6.35, 26.7081) -> (6.35, 26.6319) centre (6.35, 26.67) ccw
  arc A93 (8.636, 26.6319) -> (8.636, 26.7081) centre (8.636, 26.67) ccw
  line L44 (22.6695, 23.5585) -> (22.987, 23.8125)
  arc A94 (23.0068, 23.7877) -> (22.9672, 23.8373) centre (22.987, 23.8125) ccw
  arc A95 (22.6497, 23.5833) -> (22.6893, 23.5337) centre (22.6695, 23.5585) ccw
  line L45 (22.987, 23.8125) -> (22.987, 22.6695)
  arc A96 (22.9553, 22.6695) -> (23.0188, 22.6695) centre (22.987, 22.6695) ccw
  arc A97 (23.0188, 23.8125) -> (22.9553, 23.8125) centre (22.987, 23.8125) ccw
  line L46 (22.6695, 22.6695) -> (23.3045, 22.6695)
  arc A98 (23.3045, 22.6378) -> (23.3045, 22.7012) centre (23.3045, 22.6695) ccw
  arc A99 (22.6695, 22.7012) -> (22.6695, 22.6378) centre (22.6695, 22.6695) ccw
  line L47 (7.4295, 23.6855) -> (7.4295, 23.8125)
  arc A100 (7.4612, 23.8125) -> (7.3978, 23.8125) centre (7.4295, 23.8125) ccw
  arc A101 (7.3978, 23.6855) -> (7.4612, 23.6855) centre (7.4295, 23.6855) ccw
  line L48 (7.4295, 23.8125) -> (8.0645, 23.8125)
  arc A102 (8.0645, 23.7808) -> (8.0645, 23.8442) centre (8.0645, 23.8125) ccw
  arc A103 (7.4295, 23.8442) -> (7.4295, 23.7808) centre (7.4295, 23.8125) ccw
  line L49 (8.0645, 23.8125) -> (7.747, 22.6695)
  arc A104 (7.7164, 22.678) -> (7.7776, 22.661) centre (7.747, 22.6695) ccw
  arc A105 (8.0951, 23.804) -> (8.0339, 23.821) centre (8.0645, 23.8125) ccw
  line L50 (44.831, 26.67) -> (44.831, 24.13)
  arc A106 (44.7929, 24.13) -> (44.8691, 24.13) centre (44.831, 24.13) ccw
  arc A107 (44.8691, 26.67) -> (44.7929, 26.67) centre (44.831, 26.67) ccw
  line L51 (44.831, 24.13) -> (47.117, 24.13)
  arc A108 (47.117, 24.0919) -> (47.117, 24.1681) centre (47.117, 24.13) ccw
  arc A109 (44.831, 24.1681) -> (44.831, 24.0919) centre (44.831, 24.13) ccw
  line L52 (47.117, 24.13) -> (47.371, 24.384)
  arc A110 (47.3979, 24.3571) -> (47.3441, 24.4109) centre (47.371, 24.384) ccw
  arc A111 (47.0901, 24.1569) -> (47.1439, 24.1031) centre (47.117, 24.13) ccw
  line L53 (47.371, 24.384) -> (47.625, 24.13)
  arc A112 (47.5981, 24.1031) -> (47.6519, 24.1569) centre (47.625, 24.13) ccw
  arc A113 (47.3979, 24.4109) -> (47.3441, 24.3571) centre (47.371, 24.384) ccw
  arc A114 (49.657, 24.0919) -> (49.657, 24.1681) centre (49.657, 24.13) ccw
  arc A115 (47.625, 24.1681) -> (47.625, 24.0919) centre (47.625, 24.13) ccw
  line L54 (49.657, 24.13) -> (49.911, 24.384)
  arc A116 (49.9379, 24.3571) -> (49.8841, 24.4109) centre (49.911, 24.384) ccw
  arc A117 (49.6301, 24.1569) -> (49.6839, 24.1031) centre (49.657, 24.13) ccw
  line L55 (49.911, 24.384) -> (50.165, 24.13)
  arc A118 (50.1381, 24.1031) -> (50.1919, 24.1569) centre (50.165, 24.13) ccw
  arc A119 (49.9379, 24.4109) -> (49.8841, 24.3571) centre (49.911, 24.384) ccw
  line L56 (50.165, 24.13) -> (52.197, 24.13)
  arc A120 (52.197, 24.0919) -> (52.197, 24.1681) centre (52.197, 24.13) ccw
  arc A121 (50.165, 24.1681) -> (50.165, 24.0919) centre (50.165, 24.13) ccw
  line L57 (52.197, 24.13) -> (52.451, 24.384)
  arc A122 (52.4779, 24.3571) -> (52.4241, 24.4109) centre (52.451, 24.384) ccw
  arc A123 (52.1701, 24.1569) -> (52.2239, 24.1031) centre (52.197, 24.13) ccw
  line L58 (52.451, 24.384) -> (52.705, 24.13)
  arc A124 (52.6781, 24.1031) -> (52.7319, 24.1569) centre (52.705, 24.13) ccw
  arc A125 (52.4779, 24.4109) -> (52.4241, 24.3571) centre (52.451, 24.384) ccw
  line L59 (52.705, 24.13) -> (54.737, 24.13)
  arc A126 (54.737, 24.0919) -> (54.737, 24.1681) centre (54.737, 24.13) ccw
  arc A127 (52.705, 24.1681) -> (52.705, 24.0919) centre (52.705, 24.13) ccw
  line L60 (54.737, 24.13) -> (54.991, 24.384)
  arc A128 (55.0179, 24.3571) -> (54.9641, 24.4109) centre (54.991, 24.384) ccw
  arc A129 (54.7101, 24.1569) -> (54.7639, 24.1031) centre (54.737, 24.13) ccw
  line L61 (54.991, 24.384) -> (55.245, 24.13)
  arc A130 (55.2181, 24.1031) -> (55.2719, 24.1569) centre (55.245, 24.13) ccw
  arc A131 (55.0179, 24.4109) -> (54.9641, 24.3571) centre (54.991, 24.384) ccw
  line L62 (55.245, 24.13) -> (57.531, 24.13)
  arc A132 (57.531, 24.0919) -> (57.531, 24.1681) centre (57.531, 24.13) ccw
  arc A133 (55.245, 24.1681) -> (55.245, 24.0919) centre (55.245, 24.13) ccw
  line L63 (57.531, 24.13) -> (57.531, 26.67)
  arc A134 (57.5691, 26.67) -> (57.4929, 26.67) centre (57.531, 26.67) ccw
  arc A135 (57.4929, 24.13) -> (57.5691, 24.13) centre (57.531, 24.13) ccw
  line L64 (57.531, 26.67) -> (55.245, 26.67)
  arc A136 (55.245, 26.7081) -> (55.245, 26.6319) centre (55.245, 26.67) ccw
  arc A137 (57.531, 26.6319) -> (57.531, 26.7081) centre (57.531, 26.67) ccw
  line L65 (55.245, 26.67) -> (54.991, 26.416)
  arc A138 (54.9641, 26.4429) -> (55.0179, 26.3891) centre (54.991, 26.416) ccw
  arc A139 (55.2719, 26.6431) -> (55.2181, 26.6969) centre (55.245, 26.67) ccw
  line L66 (54.991, 26.416) -> (54.737, 26.67)
  arc A140 (54.7639, 26.6969) -> (54.7101, 26.6431) centre (54.737, 26.67) ccw
  arc A141 (54.9641, 26.3891) -> (55.0179, 26.4429) centre (54.991, 26.416) ccw
  line L67 (54.737, 26.67) -> (52.705, 26.67)
  arc A142 (52.705, 26.7081) -> (52.705, 26.6319) centre (52.705, 26.67) ccw
  arc A143 (54.737, 26.6319) -> (54.737, 26.7081) centre (54.737, 26.67) ccw
  line L68 (52.705, 26.67) -> (52.451, 26.416)
  arc A144 (52.4241, 26.4429) -> (52.4779, 26.3891) centre (52.451, 26.416) ccw
  arc A145 (52.7319, 26.6431) -> (52.6781, 26.6969) centre (52.705, 26.67) ccw
  line L69 (52.451, 26.416) -> (52.197, 26.67)
  arc A146 (52.2239, 26.6969) -> (52.1701, 26.6431) centre (52.197, 26.67) ccw
  arc A147 (52.4241, 26.3891) -> (52.4779, 26.4429) centre (52.451, 26.416) ccw
  line L70 (52.197, 26.67) -> (50.165, 26.67)
  arc A148 (50.165, 26.7081) -> (50.165, 26.6319) centre (50.165, 26.67) ccw
  arc A149 (52.197, 26.6319) -> (52.197, 26.7081) centre (52.197, 26.67) ccw
  line L71 (50.165, 26.67) -> (49.911, 26.416)
  arc A150 (49.8841, 26.4429) -> (49.9379, 26.3891) centre (49.911, 26.416) ccw
  arc A151 (50.1919, 26.6431) -> (50.1381, 26.6969) centre (50.165, 26.67) ccw
  line L72 (49.911, 26.416) -> (49.657, 26.67)
  arc A152 (49.6839, 26.6969) -> (49.6301, 26.6431) centre (49.657, 26.67) ccw
  arc A153 (49.8841, 26.3891) -> (49.9379, 26.4429) centre (49.911, 26.416) ccw
  line L73 (49.657, 26.67) -> (47.625, 26.67)
  arc A154 (47.625, 26.7081) -> (47.625, 26.6319) centre (47.625, 26.67) ccw
  arc A155 (49.657, 26.6319) -> (49.657, 26.7081) centre (49.657, 26.67) ccw
  line L74 (47.625, 26.67) -> (47.371, 26.416)
  arc A156 (47.3441, 26.4429) -> (47.3979, 26.3891) centre (47.371, 26.416) ccw
  arc A157 (47.6519, 26.6431) -> (47.5981, 26.6969) centre (47.625, 26.67) ccw
  line L75 (47.371, 26.416) -> (47.117, 26.67)
  arc A158 (47.1439, 26.6969) -> (47.0901, 26.6431) centre (47.117, 26.67) ccw
  arc A159 (47.3441, 26.3891) -> (47.3979, 26.4429) centre (47.371, 26.416) ccw
  line L76 (47.117, 26.67) -> (44.831, 26.67)
  arc A160 (44.831, 26.7081) -> (44.831, 26.6319) centre (44.831, 26.67) ccw
  arc A161 (47.117, 26.6319) -> (47.117, 26.7081) centre (47.117, 26.67) ccw
  line L77 (43.7515, 25.7175) -> (44.069, 25.9715)
  arc A162 (44.0888, 25.9467) -> (44.0492, 25.9963) centre (44.069, 25.9715) ccw
  arc A163 (43.7317, 25.7423) -> (43.7713, 25.6927) centre (43.7515, 25.7175) ccw
  line L78 (44.069, 25.9715) -> (44.069, 24.8285)
  arc A164 (44.0373, 24.8285) -> (44.1008, 24.8285) centre (44.0691, 24.8285) ccw
  arc A165 (44.1008, 25.9715) -> (44.0373, 25.9715) centre (44.0691, 25.9715) ccw
  line L79 (43.7515, 24.8285) -> (44.3865, 24.8285)
  arc A166 (44.3865, 24.7968) -> (44.3865, 24.8603) centre (44.3865, 24.8286) ccw
  arc A167 (43.7515, 24.8603) -> (43.7515, 24.7968) centre (43.7515, 24.8286) ccw
  line L80 (57.8485, 24.8285) -> (58.2295, 24.8285)
  arc A168 (58.2295, 24.7968) -> (58.2295, 24.8603) centre (58.2295, 24.8286) ccw
  arc A169 (57.8485, 24.8603) -> (57.8485, 24.7968) centre (57.8485, 24.8286) ccw
  arc A170 (58.2295, 24.8285) -> (58.4835, 25.0825) centre (58.2295, 25.0825) ccw
  arc A171 (58.2295, 24.8603) -> (58.2295, 24.7968) centre (58.2295, 24.8286) ccw
  arc A172 (58.5153, 25.0825) -> (58.4517, 25.0825) centre (58.4835, 25.0825) ccw
  line L81 (58.4835, 25.0825) -> (58.4835, 25.2095)
  arc A173 (58.5153, 25.2095) -> (58.4517, 25.2095) centre (58.4835, 25.2095) ccw
  arc A174 (58.4517, 25.0825) -> (58.5153, 25.0825) centre (58.4835, 25.0825) ccw
  arc A175 (58.4835, 25.2095) -> (58.2295, 25.4635) centre (58.2295, 25.2095) ccw
  arc A176 (58.4517, 25.2095) -> (58.5153, 25.2095) centre (58.4835, 25.2095) ccw
  arc A177 (58.2295, 25.4952) -> (58.2295, 25.4318) centre (58.2295, 25.4635) ccw
  line L82 (58.2295, 25.4635) -> (57.8485, 25.4635)
  arc A178 (57.8485, 25.4952) -> (57.8485, 25.4318) centre (57.8485, 25.4635) ccw
  arc A179 (58.2295, 25.4318) -> (58.2295, 25.4952) centre (58.2295, 25.4635) ccw
  line L83 (57.8485, 25.4635) -> (57.8485, 25.9715)
  arc A180 (57.8803, 25.9715) -> (57.8167, 25.9715) centre (57.8485, 25.9715) ccw
  arc A181 (57.8167, 25.4635) -> (57.8803, 25.4635) centre (57.8485, 25.4635) ccw
  line L84 (57.8485, 25.9715) -> (58.4835, 25.9715)
  arc A182 (58.4835, 25.9398) -> (58.4835, 26.0033) centre (58.4835, 25.9716) ccw
  arc A183 (57.8485, 26.0033) -> (57.8485, 25.9398) centre (57.8485, 25.9716) ccw
  arc A184 (54.2831, 60.3771) -> (56.2831, 60.3771) centre (55.2831, 60.3771) ccw
  arc A185 (54.3149, 60.3771) -> (54.2514, 60.3771) centre (54.2832, 60.3771) ccw
  arc A186 (56.3149, 60.3771) -> (56.2514, 60.3771) centre (56.2832, 60.3771) ccw
  line L85 (49.7229, 54.6302) -> (49.9839, 54.839)
  arc A187 (49.9958, 54.8241) -> (49.972, 54.8539) centre (49.9839, 54.839) ccw
  arc A188 (49.711, 54.645) -> (49.7348, 54.6153) centre (49.7229, 54.6302) ccw
  line L86 (49.9839, 54.839) -> (49.9839, 53.8992)
  arc A189 (49.9649, 53.8992) -> (50.003, 53.8992) centre (49.984, 53.8992) ccw
  arc A190 (50.003, 54.839) -> (49.9649, 54.839) centre (49.984, 54.839) ccw
  line L87 (49.7229, 53.8992) -> (50.245, 53.8992)
  arc A191 (50.245, 53.8802) -> (50.245, 53.9183) centre (50.245, 53.8993) ccw
  arc A192 (49.7229, 53.9183) -> (49.7229, 53.8802) centre (49.7229, 53.8993) ccw
  arc A193 (53.245, 49.6041) -> (53.01, 49.839) centre (53.01, 49.604) ccw
  arc A194 (53.226, 49.6041) -> (53.2641, 49.6041) centre (53.2451, 49.6041) ccw
  arc A195 (53.01, 49.8581) -> (53.01, 49.82) centre (53.01, 49.8391) ccw
  arc A196 (53.01, 49.839) -> (52.7229, 49.6302) centre (53.01, 49.5372) ccw
  arc A197 (53.0101, 49.82) -> (53.01, 49.858) centre (53.0101, 49.839) ccw
  arc A198 (52.7048, 49.636) -> (52.741, 49.6243) centre (52.7229, 49.6302) ccw
  arc A199 (53.1667, 49.4213) -> (53.245, 49.6041) centre (52.9925, 49.6041) ccw
  arc A200 (53.1535, 49.4351) -> (53.1798, 49.4075) centre (53.1667, 49.4213) ccw
  arc A201 (53.264, 49.604) -> (53.226, 49.6041) centre (53.245, 49.6041) ccw
  line L88 (53.1667, 49.4213) -> (52.7229, 48.8992)
  arc A202 (52.7084, 48.9115) -> (52.7374, 48.8869) centre (52.7229, 48.8992) ccw
  arc A203 (53.1812, 49.409) -> (53.1522, 49.4336) centre (53.1667, 49.4213) ccw
  line L89 (52.7229, 48.8992) -> (53.245, 48.8992)
  arc A204 (53.245, 48.8802) -> (53.245, 48.9183) centre (53.245, 48.8993) ccw
  arc A205 (52.7229, 48.9183) -> (52.7229, 48.8802) centre (52.7229, 48.8993) ccw
  line L90 (55.7229, 53.8992) -> (55.9839, 53.8992)
  arc A206 (55.9839, 53.8802) -> (55.9839, 53.9183) centre (55.9839, 53.8993) ccw
  arc A207 (55.7229, 53.9183) -> (55.7229, 53.8802) centre (55.7229, 53.8993) ccw
  arc A208 (55.9839, 53.8992) -> (55.9839, 54.4213) centre (55.9839, 54.1603) ccw
  arc A209 (55.9839, 53.9183) -> (55.9839, 53.8802) centre (55.9839, 53.8993) ccw
  arc A210 (55.9839, 54.4404) -> (55.9839, 54.4023) centre (55.9839, 54.4214) ccw
  line L91 (55.7229, 54.839) -> (56.0362, 54.839)
  arc A211 (56.0362, 54.82) -> (56.0362, 54.8581) centre (56.0362, 54.8391) ccw
  arc A212 (55.7229, 54.8581) -> (55.7229, 54.82) centre (55.7229, 54.8391) ccw
  arc A213 (56.0362, 54.4213) -> (56.0362, 54.839) centre (56.0362, 54.6302) ccw
  arc A214 (56.0362, 54.4404) -> (56.0362, 54.4023) centre (56.0362, 54.4214) ccw
  arc A215 (56.0362, 54.8581) -> (56.0362, 54.82) centre (56.0362, 54.8391) ccw
  line L92 (56.0362, 54.4213) -> (55.8273, 54.4213)
  arc A216 (55.8273, 54.4404) -> (55.8273, 54.4023) centre (55.8273, 54.4214) ccw
  arc A217 (56.0362, 54.4023) -> (56.0362, 54.4404) centre (56.0362, 54.4214) ccw
  arc A218 (55.2831, 45.8771) -> (55.2831, 61.8771) centre (55.2831, 53.8771) ccw
  arc A219 (55.2831, 61.8771) -> (55.2831, 45.8771) centre (55.2831, 53.8771) ccw
  arc A220 (55.2831, 47.3579) -> (55.2831, 60.3963) centre (55.2831, 53.8771) ccw
  arc A221 (55.2831, 60.3963) -> (55.2831, 47.3579) centre (55.2831, 53.8771) ccw
  arc A222 (55.2831, 44.3771) -> (55.2831, 63.3771) centre (55.2831, 53.8771) ccw
  arc A223 (55.2831, 63.3771) -> (55.2831, 44.3771) centre (55.2831, 53.8771) ccw
  arc A224 (54.2196, 81.5062) -> (56.2196, 81.5062) centre (55.2196, 81.5062) ccw
  arc A225 (54.2514, 81.5062) -> (54.1878, 81.5062) centre (54.2196, 81.5062) ccw
  arc A226 (56.2514, 81.5062) -> (56.1878, 81.5062) centre (56.2196, 81.5062) ccw
  line L93 (49.6594, 75.7593) -> (49.9204, 75.9681)
  arc A227 (49.9323, 75.9532) -> (49.9085, 75.983) centre (49.9204, 75.9681) ccw
  arc A228 (49.6475, 75.7741) -> (49.6713, 75.7444) centre (49.6594, 75.7593) ccw
  line L94 (49.9204, 75.9681) -> (49.9204, 75.0283)
  arc A229 (49.9014, 75.0283) -> (49.9395, 75.0283) centre (49.9205, 75.0283) ccw
  arc A230 (49.9395, 75.9681) -> (49.9014, 75.9681) centre (49.9205, 75.9681) ccw
  line L95 (49.6594, 75.0283) -> (50.1815, 75.0283)
  arc A231 (50.1815, 75.0093) -> (50.1815, 75.0473) centre (50.1815, 75.0283) ccw
  arc A232 (49.6594, 75.0473) -> (49.6594, 75.0093) centre (49.6594, 75.0283) ccw
  arc A233 (53.1815, 70.7332) -> (52.9466, 70.9681) centre (52.9466, 70.7332) ccw
  arc A234 (53.1624, 70.7332) -> (53.2005, 70.7332) centre (53.1815, 70.7332) ccw
  arc A235 (52.9466, 70.9871) -> (52.9466, 70.9491) centre (52.9466, 70.9681) ccw
  arc A236 (52.9466, 70.9681) -> (52.6594, 70.7593) centre (52.9466, 70.6663) ccw
  arc A237 (52.9466, 70.9491) -> (52.9465, 70.9871) centre (52.9466, 70.9681) ccw
  arc A238 (52.6413, 70.7651) -> (52.6775, 70.7534) centre (52.6594, 70.7593) ccw
  arc A239 (53.1032, 70.5504) -> (53.1815, 70.7332) centre (52.929, 70.7332) ccw
  arc A240 (53.09, 70.5642) -> (53.1163, 70.5366) centre (53.1031, 70.5504) ccw
  arc A241 (53.2005, 70.7331) -> (53.1625, 70.7332) centre (53.1815, 70.7332) ccw
  line L96 (53.1032, 70.5504) -> (52.6594, 70.0283)
  arc A242 (52.6449, 70.0406) -> (52.6739, 70.016) centre (52.6594, 70.0283) ccw
  arc A243 (53.1177, 70.5381) -> (53.0887, 70.5627) centre (53.1032, 70.5504) ccw
  line L97 (52.6594, 70.0283) -> (53.1815, 70.0283)
  arc A244 (53.1815, 70.0093) -> (53.1815, 70.0473) centre (53.1815, 70.0283) ccw
  arc A245 (52.6594, 70.0473) -> (52.6594, 70.0093) centre (52.6594, 70.0283) ccw
  line L98 (55.6594, 75.0283) -> (55.9204, 75.0283)
  arc A246 (55.9204, 75.0093) -> (55.9204, 75.0473) centre (55.9204, 75.0283) ccw
  arc A247 (55.6594, 75.0473) -> (55.6594, 75.0093) centre (55.6594, 75.0283) ccw
  arc A248 (55.9204, 75.0283) -> (55.9204, 75.5504) centre (55.9204, 75.2894) ccw
  arc A249 (55.9204, 75.0473) -> (55.9204, 75.0093) centre (55.9204, 75.0283) ccw
  arc A250 (55.9204, 75.5695) -> (55.9204, 75.5314) centre (55.9204, 75.5505) ccw
  line L99 (55.6594, 75.9681) -> (55.9727, 75.9681)
  arc A251 (55.9727, 75.9491) -> (55.9727, 75.9871) centre (55.9727, 75.9681) ccw
  arc A252 (55.6594, 75.9871) -> (55.6594, 75.9491) centre (55.6594, 75.9681) ccw
  arc A253 (55.9727, 75.5504) -> (55.9727, 75.9681) centre (55.9727, 75.7593) ccw
  arc A254 (55.9727, 75.5695) -> (55.9727, 75.5314) centre (55.9727, 75.5505) ccw
  arc A255 (55.9727, 75.9871) -> (55.9727, 75.9491) centre (55.9727, 75.9681) ccw
  line L100 (55.9727, 75.5504) -> (55.7638, 75.5504)
  arc A256 (55.7638, 75.5695) -> (55.7638, 75.5314) centre (55.7638, 75.5505) ccw
  arc A257 (55.9727, 75.5314) -> (55.9727, 75.5695) centre (55.9727, 75.5505) ccw
  arc A258 (55.2196, 67.0062) -> (55.2196, 83.0062) centre (55.2196, 75.0062) ccw
  arc A259 (55.2196, 83.0062) -> (55.2196, 67.0062) centre (55.2196, 75.0062) ccw
  arc A260 (55.2196, 68.487) -> (55.2196, 81.5254) centre (55.2196, 75.0062) ccw
  arc A261 (55.2196, 81.5254) -> (55.2196, 68.487) centre (55.2196, 75.0062) ccw
  arc A262 (55.2196, 65.5062) -> (55.2196, 84.5062) centre (55.2196, 75.0062) ccw
  arc A263 (55.2196, 84.5062) -> (55.2196, 65.5062) centre (55.2196, 75.0062) ccw
  arc A264 (97.4424, 18.6412) -> (99.4424, 18.6412) centre (98.4424, 18.6412) ccw
  arc A265 (97.4741, 18.6412) -> (97.4106, 18.6412) centre (97.4424, 18.6412) ccw
  arc A266 (99.4741, 18.6412) -> (99.4106, 18.6412) centre (99.4424, 18.6412) ccw
  line L101 (94.8822, 15.8943) -> (95.1432, 16.1031)
  arc A267 (95.1551, 16.0882) -> (95.1313, 16.118) centre (95.1432, 16.1031) ccw
  arc A268 (94.8703, 15.9091) -> (94.8941, 15.8794) centre (94.8822, 15.8943) ccw
  line L102 (95.1432, 16.1031) -> (95.1432, 15.1633)
  arc A269 (95.1242, 15.1633) -> (95.1623, 15.1633) centre (95.1432, 15.1633) ccw
  arc A270 (95.1623, 16.1031) -> (95.1242, 16.1031) centre (95.1432, 16.1031) ccw
  line L103 (94.8822, 15.1633) -> (95.4043, 15.1633)
  arc A271 (95.4043, 15.1443) -> (95.4043, 15.1824) centre (95.4043, 15.1633) ccw
  arc A272 (94.8822, 15.1824) -> (94.8822, 15.1443) centre (94.8822, 15.1633) ccw
  arc A273 (101.4043, 15.8681) -> (101.1693, 16.1031) centre (101.1693, 15.8681) ccw
  arc A274 (101.3852, 15.8681) -> (101.4233, 15.8681) centre (101.4043, 15.8681) ccw
  arc A275 (101.1693, 16.1222) -> (101.1693, 16.0841) centre (101.1693, 16.1031) ccw
  arc A276 (101.1693, 16.1031) -> (100.8822, 15.8943) centre (101.1693, 15.8013) ccw
  arc A277 (101.1693, 16.0841) -> (101.1693, 16.1221) centre (101.1693, 16.1031) ccw
  arc A278 (100.864, 15.9001) -> (100.9003, 15.8884) centre (100.8821, 15.8943) ccw
  arc A279 (101.326, 15.6854) -> (101.4043, 15.8681) centre (101.1519, 15.8681) ccw
  arc A280 (101.3128, 15.6992) -> (101.3391, 15.6716) centre (101.326, 15.6854) ccw
  arc A281 (101.4233, 15.8681) -> (101.3852, 15.8682) centre (101.4043, 15.8682) ccw
  line L104 (101.326, 15.6854) -> (100.8822, 15.1633)
  arc A282 (100.8677, 15.1756) -> (100.8967, 15.151) centre (100.8822, 15.1633) ccw
  arc A283 (101.3405, 15.6731) -> (101.3114, 15.6977) centre (101.326, 15.6854) ccw
  line L105 (100.8822, 15.1633) -> (101.4043, 15.1633)
  arc A284 (101.4043, 15.1443) -> (101.4043, 15.1824) centre (101.4043, 15.1633) ccw
  arc A285 (100.8822, 15.1824) -> (100.8822, 15.1443) centre (100.8822, 15.1633) ccw
  arc A286 (98.4424, 4.1412) -> (98.4424, 20.1412) centre (98.4424, 12.1412) ccw
  arc A287 (98.4424, 20.1412) -> (98.4424, 4.1412) centre (98.4424, 12.1412) ccw
  arc A288 (98.4424, 5.622) -> (98.4424, 18.6604) centre (98.4424, 12.1412) ccw
  arc A289 (98.4424, 18.6604) -> (98.4424, 5.622) centre (98.4424, 12.1412) ccw
  arc A290 (98.4424, 2.6412) -> (98.4424, 21.6412) centre (98.4424, 12.1412) ccw
  arc A291 (98.4424, 21.6412) -> (98.4424, 2.6412) centre (98.4424, 12.1412) ccw
  arc A292 (97.4358, 39.2896) -> (99.4358, 39.2896) centre (98.4358, 39.2896) ccw
  arc A293 (97.4675, 39.2896) -> (97.404, 39.2896) centre (97.4357, 39.2896) ccw
  arc A294 (99.4675, 39.2896) -> (99.404, 39.2896) centre (99.4358, 39.2896) ccw
  line L106 (94.8756, 36.5427) -> (95.1366, 36.7515)
  arc A295 (95.1485, 36.7367) -> (95.1247, 36.7664) centre (95.1366, 36.7515) ccw
  arc A296 (94.8637, 36.5576) -> (94.8875, 36.5278) centre (94.8756, 36.5427) ccw
  line L107 (95.1366, 36.7515) -> (95.1366, 35.8117)
  arc A297 (95.1176, 35.8117) -> (95.1557, 35.8117) centre (95.1367, 35.8117) ccw
  arc A298 (95.1557, 36.7515) -> (95.1176, 36.7515) centre (95.1367, 36.7515) ccw
  line L108 (94.8756, 35.8117) -> (95.3977, 35.8117)
  arc A299 (95.3977, 35.7927) -> (95.3977, 35.8308) centre (95.3977, 35.8118) ccw
  arc A300 (94.8756, 35.8308) -> (94.8756, 35.7927) centre (94.8756, 35.8118) ccw
  arc A301 (101.3977, 36.5166) -> (101.1627, 36.7515) centre (101.1627, 36.5165) ccw